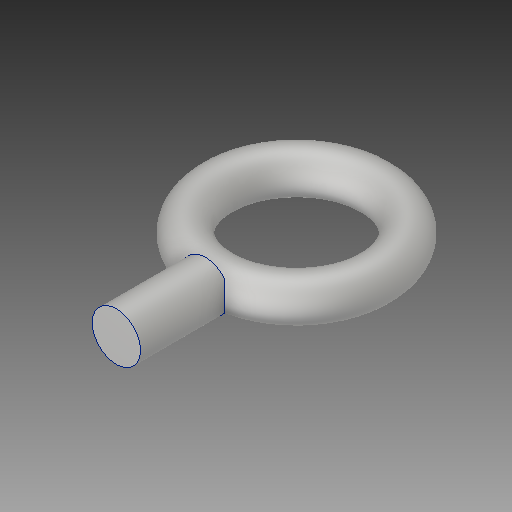
# Autodesk Inventor part: 24mm ID Eye bolt
Saved by Autodesk Inventor 2019 (Build 230136000, 136)
## iProperties
Created: 2019-11-03
Part Number: 24mm ID Eye bolt
Material: Aluminum 6061
Document SubType Name: Modeling
Designer: admin
Density: 2.7 g/cm^3
Appearance: Aluminum - Flat
Author: admin
Autodesk Inventor part; units mm, degrees
ref_plane "YZ Plane" through (0, 0, 0) normal (1, 0, 0) x (0, 1, 0)
ref_plane "XZ Plane" through (0, 0, 0) normal (0, 1, 0) x (-1, 0, 0)
ref_plane "XY Plane" through (0, 0, 0) normal (0, 0, 1) x (1, 0, 0)
sketch "Sketch1" plane through (0, 0, 0) normal (0, 0, 1) x (1, 0, 0)
  circle A0 centre (16.305, 0) radius 4.245
  line L0 (16.305, 0) -> (0, 0) construction
  line L1 (0, 0) -> (0, -5.537) construction
  dimension "d0" = 8.49
  dimension "d1" = 16.305
  constraints: 4 end point, 1 centre point, 1 horizontal, 1 vertical
  measures "d0" diameter of A0
  measures "d1" distance of L0.start L0.end
revolve "Revolution1" add sketch "Sketch1" angle 360 about axis through (0, 0, 0) along (0, -1, 0)
sketch "Sketch2" plane through (0, 0, 0) normal (0, 1, 0) x (-1, 0, 0)
  line L0 (5, 18.8631) -> (0, 18.8631)
  line L1 (0, 18.8631) -> (0, 37.3631)
  line L2 (0, 37.3631) -> (5, 37.3631)
  line L3 (5, 37.3631) -> (5, 18.8631)
  point P0 (0, 0)
  dimension "d3" = 5
  dimension "d4" = 18.5
  constraints: 8 end point, 2 parallel, 1 horizontal, 1 perpendicular, 1 point on line
  measures "d3" distance of L1.end L2.end
  measures "d4" distance of L0.end L1.end
revolve "Revolution2" add sketch "Sketch2" angle 360 about axis through (0, 0, 18.8631) along (0, 0, 1)
body "Solid1"
